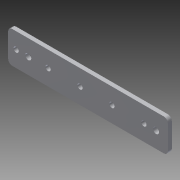
# Autodesk Inventor part: Spacer for Belt
Saved by Autodesk Inventor 2014 (Build 180170000, 170)
## iProperties
Created: 2014-01-22
Part Number: Spacer for Belt
Material: Aluminum 6061
Document SubType Name: Modeling
Designer: Michael
Density: 2.71 g/cm^3
Appearance: Aluminum - Flat
Author: Michael
Autodesk Inventor part; units mm, degrees
ref_plane "YZ Plane" through (0, 0, 0) normal (1, 0, 0) x (0, 1, 0)
ref_plane "XZ Plane" through (0, 0, 0) normal (0, 1, 0) x (-1, 0, 0)
ref_plane "XY Plane" through (0, 0, 0) normal (0, 0, 1) x (1, 0, 0)
sketch "Sketch1" plane through (0, 0, 0) normal (0, 0, 1) x (1, 0, 0)
  line L0 (0, 0) -> (127, 0)
  line L1 (127, 0) -> (127, 25.4)
  line L2 (127, 25.4) -> (0, 25.4)
  line L3 (0, 25.4) -> (0, 0)
  circle A0 centre (6.35, 12.7) radius 2.0701
  circle A1 centre (31.75, 12.7) radius 2.0701
  circle A2 centre (57.15, 12.7) radius 2.0701
  circle A3 centre (82.55, 12.7) radius 2.0701
  circle A4 centre (107.95, 12.7) radius 2.0701
  circle A5 centre (117.602, 12.7) radius 2.413
  circle A6 centre (16.002, 12.7) radius 2.413
  dimension "d0" = 127
  dimension "d1" = 25.4
  dimension "d2" = 4.1402
  dimension "d3" = 12.7
  dimension "d4" = 6.35
  dimension "d7" = 25.4
  dimension "d12" = 4.826
  dimension "d15" = 101.6
  dimension "d21" = 9.652
  dimension "d22" = 12.7
  constraints: 8 end point, 7 centre point, 3 horizontal, 2 parallel, 1 perpendicular, 10 other
  measures "d0" distance of L2.end L1.end
  measures "d1" distance of L1.end L0.end
  measures "d2" diameter of A0
  measures "d3" distance from line of L0 A0.centre
  measures "d4" distance from line of L3 A0.centre
  measures "d7" distance of A0.centre A1.centre
  measures "d12" diameter of A5
  measures "d15" distance of A5.centre A6.centre
  measures "d21" distance of A4.centre A5.centre
  measures "d22" distance from line of L0 A5.centre
extrude "Extrusion1" add sketch "Sketch1" along normal blind 3.175
fillet "Fillet1" radius 3.175 4 edges at (0, 25.4, 1.5875) (127, 25.4, 1.5875) (127, 0, 1.5875) (0, 0, 1.5875)
body "Solid1"
